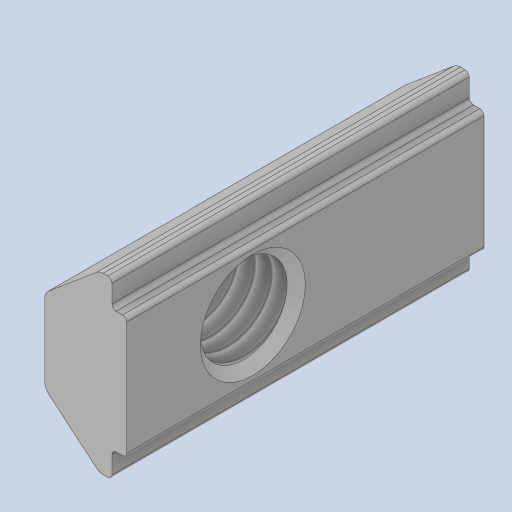
# Autodesk Inventor part: HNTP5-5
Saved by Autodesk Inventor 2023 (Build 270158000, 158)
## iProperties
Created: 2023-10-30
Part Number: HNTP5-5
Material: Generic
Catalog Web Link: www.cadenas.de
Description: HNTP5, HNTPV5, HNTPZ5, SHNTP5-Post-Assembly Insertion Nuts with Spring Stoppers For HFS5 Series Aluminum Extrusions 20, 25, 40 Square
Vendor: MISUMI
Document SubType Name: Modeling
Designer: psAdmin
Manufacturer: MISUMI
Mass: 0.370869 g
Surface Area: 4.44 cm^2
Volume: 0.370869 cm^3
Density: 1 g/cm^3
Appearance: PSOLRGB-175-175-175
Category: PARTsolutions
Company: MISUMI
PSOL_IDENT_0: {$CADENAS_DATA/23d-libs/misumi/metric/38_al_extrusions_blackets/nuts/hntp5.prj},179 {VTYP=3D},{NB=HN
PSOL_IDENT_1: TP5-5},{LINA=HNTP5-5},{NN=HNTP5, HNTPV5, HNTPZ5, SHNTP5},{DATE=16.05.2023 02:28:52},{GEOMDATE=05.11.
PSOL_IDENT_2: 2019 06:59:09},{VERSION=},{LINEID=10},{WBVAR=M},{WBNUMERIC=M}  {NB=HNTP5-5},{LINA=HNTP5-5},{KT=DUMMY
PSOL_IDENT_3: },{PN=HNTP5-5},{TYPE=HNTP},{TS=1010 Carbon Steel Equivalent},{TSALG=HNTP},{M=5},{MALG=3,4,5},{L1=6.0
PSOL_IDENT_4: }
NB: HNTP5-5
NN: HNTP5, HNTPV5, HNTPZ5, SHNTP5
NT: Post-Assembly Insertion Nuts with Spring Stoppers For HFS5 Series Aluminum Extrusions 20, 25, 40 Square
NBSYN: $PN.
LINA: HNTP5-5
CATALOG: Misumi
PN: HNTP5-5
TS: 1010 Carbon Steel Equivalent
M: 5
L1: 6
SUPPLIER: MISUMI
ARTICLENO: HNTP5-5
BOMINFO: HNTP5-5
CREATOR: CADENAS GmbH
Title: HNTP5-5
Author: Cadenas PARTsolutions
Comments: Post-Assembly Insertion Nuts with Spring Stoppers For HFS5 Series Aluminum Extrusions 20, 25, 40 Square
Autodesk Inventor part; units mm, degrees
sketch "_____2" plane through (0, 0, 0) normal (0, 0, 1) x (1, 0, 0)
  arc A0 (0, -1.7352) -> (0.1786, -2.1182) centre (0.5, -1.7352) ccw
  line L0 (0.1786, -2.1182) -> (2.4606, -4.033)
  arc A1 (2.4606, -4.033) -> (2.782, -4.15) centre (2.782, -3.65) ccw
  line L1 (2.782, -4.15) -> (3, -4.15)
  arc A2 (3, -4.15) -> (3.2, -3.95) centre (3, -3.95) ccw
  line L2 (3.2, -3.95) -> (3.2, -3.1)
  arc A3 (3.4, -2.9) -> (3.2, -3.1) centre (3.4, -3.1) ccw
  line L3 (3.4, -2.9) -> (3.7, -2.9)
  arc A4 (3.7, -2.9) -> (3.9, -2.7) centre (3.7, -2.7) ccw
  line L4 (3.9, -2.7) -> (3.9, 2.7)
  arc A5 (3.9, 2.7) -> (3.7, 2.9) centre (3.7, 2.7) ccw
  line L5 (3.7, 2.9) -> (3.4, 2.9)
  arc A6 (3.2, 3.1) -> (3.4, 2.9) centre (3.4, 3.1) ccw
  line L6 (3.2, 3.1) -> (3.2, 3.95)
  arc A7 (3.2, 3.95) -> (3, 4.15) centre (3, 3.95) ccw
  line L7 (3, 4.15) -> (2.782, 4.15)
  arc A8 (2.782, 4.15) -> (2.4606, 4.033) centre (2.782, 3.65) ccw
  line L8 (2.4606, 4.033) -> (0.1786, 2.1182)
  arc A9 (0.1786, 2.1182) -> (0, 1.7352) centre (0.5, 1.7352) ccw
  line L9 (0, 1.7352) -> (0, -1.7352)
  constraints: 20 end point, 20 point on circle, 10 centre point
extrude "Extrusion1" add sketch "_____2" along normal mid plane 17
sketch "Sketch_2" plane through (0, 0, 2.5) normal (0, 0, 1) x (1, 0, 0)
  line L0 (3.9, 0) -> (0, 0)
  line L1 (0, 0) -> (0, 2.5)
  line L2 (0, 2.5) -> (0.433, 2.067)
  line L3 (0.433, 2.067) -> (3.467, 2.067)
  line L4 (3.467, 2.067) -> (3.9, 2.5)
  line L5 (3.9, 2.5) -> (3.9, 0)
  line L6 (3.9, 0) -> (0, 0)
  constraints: 14 end point
revolve "Revolution1" cut sketch "Sketch_2" angle 360 about axis through (3.9, 0, 2.5) along (1, 0, 0)
thread "Thread1" size "M5x0.8" class "6H" standard "ISO Metric profile" full length
sketch "_____1" plane through (0, 0, -4.5) normal (0, 0, 1) x (1, 0, 0)
  line L0 (0.95, 0) -> (0, 0)
  line L1 (0, 0) -> (0, 1.75)
  line L2 (0, 1.75) -> (0.95, 1.75)
  line L3 (0.95, 1.75) -> (0.95, 0)
  line L4 (0.95, 0) -> (0, 0)
  constraints: 10 end point
revolve "Revolution2" cut sketch "_____1" angle 360 about axis through (0.95, 0, -4.5) along (1, 0, 0)
sketch "Sketch_3" plane through (0, 0, -4.5) normal (0, 0, 1) x (1, 0, 0)
  line L0 (2.7, 0) -> (-0.8, 0)
  arc A0 (2.7, 0) -> (-0.8, 0) centre (0.95, 0) ccw
  line L1 (2.7, 0) -> (-0.8, 0)
  constraints: 4 end point, 2 point on circle, 1 centre point
revolve "Revolution3" add sketch "Sketch_3" angle 360 about axis through (2.7, 0, -4.5) along (1, 0, 0)
ref_plane "to_blackets_XY" through (3.9, 0, 2.5) normal (1, 0, 0) x (0, 0, -1)
ref_plane "to_blackets_YZ" through (3.9, 0, 2.5) normal (0, 0, -1) x (0, 1, 0)
ref_plane "to_blackets_ZX" through (3.9, 0, 2.5) normal (0, 1, 0) x (1, 0, 0)
ref_plane "to_bolt_XY" through (0, 0, 2.5) normal (1, 0, 0) x (0, 0, -1)
ref_plane "to_bolt_YZ" through (0, 0, 2.5) normal (0, 0, -1) x (0, 1, 0)
ref_plane "to_bolt_ZX" through (0, 0, 2.5) normal (0, 1, 0) x (1, 0, 0)
ref_plane "to_frames_XY" through (3.2, 0, 2.5) normal (1, 0, 0) x (0, 0, -1)
ref_plane "to_frames_YZ" through (3.2, 0, 2.5) normal (0, 0, -1) x (0, 1, 0)
ref_plane "to_frames_ZX" through (3.2, 0, 2.5) normal (0, 1, 0) x (1, 0, 0)
body "Solid1"
